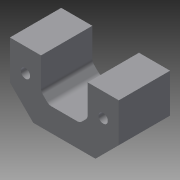
# Autodesk Inventor part: Arm_Link
Saved by Autodesk Inventor 2013 (Build 170138000, 138)
## iProperties
Created: 2014-05-07
Part Number: Arm_Link
Material: 一般
Document SubType Name: Modeling
Designer: andou
Density: 1 g/cm^3
Author: andou
Autodesk Inventor part; units mm, degrees
ref_plane "YZ Plane" through (0, 0, 0) normal (1, 0, 0) x (0, 1, 0)
ref_plane "XZ Plane" through (0, 0, 0) normal (0, 1, 0) x (-1, 0, 0)
ref_plane "XY Plane" through (0, 0, 0) normal (0, 0, 1) x (1, 0, 0)
sketch "スケッチ1" plane through (0, 0, 0) normal (0, 1, 0) x (-1, 0, 0)
  line L0 (-17.5004, 7.4992) -> (-7.5004, 7.4996)
  line L1 (-7.5004, 7.4996) -> (-7.4999, -2.5004)
  line L2 (-7.4999, -2.5004) -> (-4.9998, -5.0002)
  line L3 (-4.9998, -5.0002) -> (5.0002, -4.9998)
  line L4 (5.0002, -4.9998) -> (7.5001, -2.4996)
  line L5 (7.5001, -2.4996) -> (7.4996, 7.5004)
  line L6 (7.4996, 7.5004) -> (17.4996, 7.5008)
  circle A0 centre (-12.5, -0.0006) radius 1.5
  circle A1 centre (12.5, 0.0006) radius 1.5
  line L7 (-17.5004, 7.4992) -> (-17.4998, -5.0008)
  line L8 (-17.4998, -5.0008) -> (-9.9994, -12.5005)
  line L9 (17.4996, 7.5008) -> (17.5002, -4.9992)
  line L10 (17.5002, -4.9992) -> (10.0006, -12.4995)
  line L11 (-9.9994, -12.5005) -> (10.0006, -12.4995)
  point P0 (0, 0)
  dimension "d2" = 10
  dimension "d3" = 135
  dimension "d4" = 45
  dimension "d6" = 15
  dimension "d7" = 2.5
  dimension "d8" = 10
  dimension "d9" = 10
  dimension "d10" = 10
  dimension "d11" = 10
  dimension "d12" = 90
  dimension "d15" = 25
  dimension "d16" = 5
  dimension "d17" = 20
  dimension "d18" = 7.5
  dimension "d19" = 7.5
  dimension "d20" = 5
  dimension "d27" = 20
  dimension "d31" = 3
  dimension "d65" = 5
  dimension "d66" = 7.5
  dimension "d67" = 12.5
  constraints: 24 end point, 3 parallel, 2 centre point, 2 equal length, 1 collinear, 1 equal radius, 1 perpendicular
  measures "d2" distance of L2.end L3.end
  measures "d3" angle of L3 L2
  measures "d4" angle of L4 L3
  measures "d6" distance between parallel lines of L5 L1
  measures "d7" distance from line of L5 L3.end
  measures "d8" distance of L4.end L5.end
  measures "d9" distance of L0.end L1.end
  measures "d10" distance of L0.start L0.end
  measures "d11" distance of L5.end L6.end
  measures "d12" angle of L0 L1
  measures "d15" distance of A1.centre A0.centre
  measures "d16" distance from line of L1 A0.centre
  measures "d17" distance of L10.end L8.end
  measures "d18" distance from line of L0 A0.centre
  measures "d19" distance from line of L6 A1.centre
  measures "d20" distance from line of L9 A1.centre
  measures "d27" distance from line of L6 L10.end
  measures "d31" diameter of A1
  measures "d65" distance from line of point (0, 0) L3
  measures "d66" distance from line of L5 point (0, 0)
  measures "d67" distance of A1.centre point (0, 0)
extrude "押し出し2" add sketch "スケッチ1" along normal blind 16.5
fillet "フィレット2" radius 2 4 edges at (-5.0002, 8.25, -4.9998) (-7.5001, 8.25, -2.4996) (4.9998, 8.25, -5.0002) (7.4999, 8.25, -2.5004)
